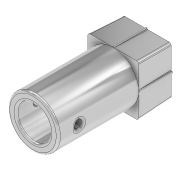
# Autodesk Inventor part: Axis 5 Drive Rod
Saved by Autodesk Inventor 2020 (Build 240168000, 168)
## iProperties
Created: 2021-06-29
Part Number: Axis 5 Drive Rod
Material: Generic
Document SubType Name: Modeling
Designer: Coy
Density: 1 g/cm^3
Appearance: Chrome - Polished
Author: Coy
Autodesk Inventor part; units mm, degrees
ref_plane "YZ Plane" through (0, 0, 0) normal (1, 0, 0) x (0, 1, 0)
ref_plane "XZ Plane" through (0, 0, 0) normal (0, 1, 0) x (-1, 0, 0)
ref_plane "XY Plane" through (0, 0, 0) normal (0, 0, 1) x (1, 0, 0)
sketch "Sketch1" plane through (0, 0, 0) normal (0, 0, 1) x (1, 0, 0)
  circle A0 centre (0, 0) radius 6
  circle A1 centre (0, 0) radius 4
  dimension "d0" = 12
  dimension "d1" = 8
  constraints: 2 centre point, 2 coincident
  measures "d0" diameter of A0
  measures "d1" diameter of A1
extrude "Extrusion1" add sketch "Sketch1" along normal blind 8.5
sketch "Sketch2" plane through (0, 0, 0) normal (0, 0, -1) x (-1, 0, 0)
  circle A0 centre (0, 0) radius 6 construction
  line L0 (-6, 6) -> (6, 6)
  line L1 (6, 6) -> (6, -6)
  line L2 (6, -6) -> (-6, -6)
  line L3 (-6, -6) -> (-6, 6)
  circle A1 centre (0, 0) radius 4 projected
  constraints: 8 end point, 2 parallel, 1 horizontal, 1 perpendicular
extrude "Extrusion2" add sketch "Sketch2" along normal blind 8
chamfer "Chamfer1" distance 8 angle 2 1 edges at (0, 6, -8) measured on face at (0, 6, -7.5)
sketch "Sketch3" plane through (0, 0, 8.5) normal (0, 0, 1) x (1, 0, 0)
  arc A0 (0.6667, 3.9441) -> (-0.6667, 3.9441) centre (0, 0) ccw projected
  circle A1 centre (0, 0) radius 4
  circle A2 centre (0, 0) radius 6
  point P0 (0.6667, 3.9441)
  dimension "d15" = 12
  constraints: 2 coincident, 1 centre point, 3 other
  measures "d15" diameter of A2
extrude "Extrusion3" add sketch "Sketch3" along normal blind 0.5
sketch "Sketch4" plane through (0, 0, 9) normal (0, 0, 1) x (1, 0, 0)
  circle A0 centre (0, 0) radius 4
  circle A1 centre (0, 0) radius 6
  dimension "d18" = 12
  dimension "d24" = 8
  constraints: 2 centre point, 2 coincident
  measures "d18" diameter of A1
  measures "d24" diameter of A0
extrude "Extrusion4" add sketch "Sketch4" along normal blind 10
sketch "Sketch5" plane through (0, 0, 0) normal (1, 0, 0) x (0, 1, 0)
  line L0 (6, -8) -> (6, 36)
  line L1 (6, 14) -> (-6, 14) construction
  line L2 (-6, -8) -> (-6, 36) construction
  circle A0 centre (0, 14) radius 1
  line L3 (6, 19) -> (-6, 19) projected
  point P0 (0, 0)
  dimension "d21" = 2
  dimension "d25" = 5
  constraints: 6 end point, 3 midpoint, 1 centre point
  measures "d21" diameter of A0
  measures "d25" distance between parallel lines of L3 L1
extrude "Extrusion5" cut sketch "Sketch5" along normal through all both and the other way through all
chamfer "Chamfer2" distance 8 angle 2 1 edges at (6, -0.1396, -8) measured on face at (6, -0.1396, -7.5)
chamfer "Chamfer3" distance 8 angle 2 1 edges at (-0.1396, -6, -8) measured on face at (-0.1396, -6, -7.5)
chamfer "Chamfer4" distance 8 angle 2 1 edges at (-6, 0, -8) measured on face at (-6, 0, -7.5)
fillet "Fillet1" radius 0.5 8 edges at (-6, 6, 0) (-5.8604, 5.8604, -4) (-6, -6, 0) (-5.8604, -5.8604, -4) (6, -6, 0) (5.8604, -5.8604, -4) (6, 6, 0) (5.8604, 5.8604, -4)
fillet "Fillet2" radius 0.5 1 edges at (4, 0, -8)
fillet "Fillet3" radius 0.5 1 edges at (-4, 0, 19)
fillet "Fillet4" radius 0.5 4 edges at (-5.9161, -1, 14.0056) (5.9539, 0.7423, 13.3299) (5.9161, -1, 14.0001) (5.9538, 0.7432, 14.6691)
sketch "Sketch6" plane through (0, 0, -8) normal (0, 0, -1) x (-1, 0, 0)
  ellipse E0 centre (-5.2203, 5.2203) end of major axis (-5.5743, 5.5743) minor radius 0.5 (-5.2209, 5.7206) -> (-5.7206, 5.2209) ccw projected
  line L0 (-5.7206, -5.2209) -> (-5.7206, 5.2209) projected
  ellipse E1 centre (-5.2203, -5.2203) end of major axis (-5.5743, -5.5743) minor radius 0.5 (-5.7206, -5.2209) -> (-5.2209, -5.7206) ccw projected
  line L1 (5.2209, -5.7206) -> (-5.2209, -5.7206) projected
  ellipse E2 centre (5.2203, -5.2203) end of major axis (5.5743, -5.5743) minor radius 0.5 (5.2209, -5.7206) -> (5.7206, -5.2209) ccw projected
  line L2 (5.7206, 5.2209) -> (5.7206, -5.2209) projected
  ellipse E3 centre (5.2203, 5.2203) end of major axis (5.5743, 5.5743) minor radius 0.5 (5.7206, 5.2209) -> (5.2209, 5.7206) ccw projected
  line L3 (-5.2209, 5.7206) -> (5.2209, 5.7206) projected
  circle A0 centre (0, 0) radius 4.5 projected
  line L4 (-5.2209, 5.7206) -> (-5.5003, 6) construction
  line L5 (-5.2209, 5.7206) -> (5.2209, 5.7206) construction
  line L6 (5.5003, 6) -> (5.2209, 5.7206) construction
  line L7 (5.5003, 6) -> (0, 6) construction
  line L8 (0, 6) -> (-5.5003, 6) construction
  line L9 (-6, 5.5003) -> (-5.7206, 5.2209) construction
  line L10 (-6, 5.5003) -> (-6, 0) construction
  line L11 (-6, 0) -> (-6, -5.5003) construction
  line L12 (-5.7206, -5.2209) -> (-6, -5.5003) construction
  line L13 (-5.7206, -5.2209) -> (-5.7206, 5.2209) construction
  line L14 (6, -5.5003) -> (5.7206, -5.2209) construction
  line L15 (6, -5.5003) -> (6, 0) construction
  line L16 (6, 0) -> (6, 5.5003) construction
  line L17 (5.7206, 5.2209) -> (6, 5.5003) construction
  line L18 (5.7206, 5.2209) -> (5.7206, -5.2209) construction
  line L19 (-5.5003, -6) -> (-5.2209, -5.7206) construction
  line L20 (-5.5003, -6) -> (0, -6) construction
  line L21 (0, -6) -> (5.5003, -6) construction
  line L22 (5.2209, -5.7206) -> (5.5003, -6) construction
  line L23 (5.2209, -5.7206) -> (-5.2209, -5.7206) construction
  line L24 (0, 6) -> (-5.5003, 6) projected
  arc A1 (0.2, 6) -> (-0.2, 6) centre (0, 6) ccw
  line L25 (-0.2, 6) -> (-0.2, 5.7206)
  line L26 (-5.2209, 5.7206) -> (5.2209, 5.7206) projected
  line L27 (5.5003, 6) -> (0, 6) projected
  line L28 (0.2, 6) -> (0.2, 5.7206)
  arc A2 (-6, 0.2) -> (-6, -0.2) centre (-6, 0) ccw
  line L29 (-6, -0.2) -> (-5.7206, -0.2)
  line L30 (-6, 0.2) -> (-5.7206, 0.2)
  arc A3 (-0.2, -6) -> (0.2, -6) centre (0, -6) ccw
  line L31 (0.2, -6) -> (0.2, -5.7206)
  line L32 (-0.2, -6) -> (-0.2, -5.7206)
  arc A4 (6, -0.2) -> (6, 0.2) centre (6, 0) ccw
  line L33 (6, 0.2) -> (5.7206, 0.2)
  line L34 (6, -0.2) -> (5.7206, -0.2)
  dimension "d39" = 0.4
  dimension "d42" = 360
  constraints: 16 end point, 8 point on circle, 4 centre point, 4 point on line, 2 perpendicular, 1 coincident, 37 other
  measures "d39" diameter of A1
extrude "Extrusion6" add sketch "Sketch6" against normal blind 8 contours L25 L24 L27 L28 L3 | L0 L29 A2 L30 | A1 L27 L24 | L33 A4 L34 L2 | L1 L31 A3 L32
fillet "Fillet5" radius 0.2 12 edges at (0.2, 5.8603, -8) (-0.2, 5.8603, -8) (0, 6.2, -8) (-5.8603, 0.2, -8) (-5.8603, -0.2, -8) (-6.2, 0, -8) (-0.2, -5.8603, -8) (0.2, -5.8603, -8) (0, -6.2, -8) (6.2, 0, -8) (5.8603, -0.2, -8) (5.8603, 0.2, -8)
fillet "Fillet6" radius 0.5 1 edges at (-6, 0, 19)
body "Solid1"
